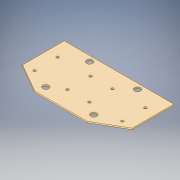
# Autodesk Inventor part: DPLX_P023 Spark Gap Shielding Bottom
Saved by Autodesk Inventor 2018 (Build 220112000, 112)
## iProperties
Created: 2017-11-28
Part Number: DPLX_P023 Spark Gap Shielding Bottom
Material: Polyethylene, High Density
Document SubType Name: Modeling
Designer: Sam
Density: 0.952 g/cm^3
Appearance: Smooth - Off-White
Mass: 11.185 g
Surface Area: 162.174 cm^2
Volume: 11.749 cm^3
Author: Sam
Comments: http://www.eplastics.com/Plastic/G9-G10-FR4-glass-epoxy-sheet/G10NAT-060X12X12
Autodesk Inventor part; units mm, degrees
ref_plane "YZ Plane" through (0, 0, 0) normal (1, 0, 0) x (0, 1, 0)
ref_plane "XZ Plane" through (0, 0, 0) normal (0, 1, 0) x (-1, 0, 0)
ref_plane "XY Plane" through (0, 0, 0) normal (0, 0, 1) x (1, 0, 0)
sketch "Sketch1" plane through (0, 0, 0) normal (0, 1, 0) x (-1, 0, 0)
  line L0 (-63.5, 33.655) -> (63.5, 33.655)
  line L1 (63.5, 33.655) -> (63.5, -33.655)
  line L2 (63.5, -33.655) -> (-63.5, -33.655)
  line L3 (-63.5, -33.655) -> (-63.5, 33.655)
  line L4 (-63.5, 33.655) -> (63.5, -33.655) construction
  line L5 (63.5, 33.655) -> (-63.5, -33.655) construction
  point P0 (0, 0)
  dimension "d0" = 127
  dimension "d1" = 67.31
  constraints: 12 end point, 2 midpoint, 2 parallel, 1 horizontal, 1 perpendicular
  measures "d0" distance of L1.end L2.end
  measures "d1" distance of L0.end L1.end
extrude "Extrusion1" add sketch "Sketch1" along normal mid plane 1.524
sketch "Sketch2" plane through (0, 0.762, 0) normal (0, 1, 0) x (1, 0, 0)
  line L0 (63.5, 33.655) -> (-63.5, 33.655) projected
  line L1 (-63.5, -33.655) -> (63.5, -33.655) projected
  line L2 (-63.5, 33.655) -> (-63.5, -33.655) projected
  line L3 (63.5, -33.655) -> (63.5, 33.655) projected
  point P0 (0, 0)
  point P1 (-50.8, 13.335)
  point P2 (-12.7, 13.335)
  point P3 (12.7, 13.335)
  point P4 (50.8, 13.335)
  point P5 (50.8, -13.335)
  point P6 (12.7, -13.335)
  point P7 (-12.7, -13.335)
  point P8 (-50.8, -13.335)
  point P9 (-50.8, -33.655)
  point P10 (50.8, -33.655)
  point P11 (-63.5, -20.955)
  point P12 (63.5, -20.955)
  dimension "d5" = 20.32
  dimension "d6" = 20.32
  dimension "d7" = 12.7
  dimension "d8" = 50.8
  dimension "d9" = 12.7
  dimension "d10" = 50.8
  constraints: 6 horizontal alignment, 4 vertical alignment
  measures "d5" distance from line of L0 point (-50.8, 13.335)
  measures "d6" distance from line of point (-50.8, -13.335) L1
  measures "d7" distance from line of L2 point (-50.8, 13.335)
  measures "d8" distance from line of point (-12.7, 13.335) L2
  measures "d9" distance from line of point (50.8, 13.335) L3
  measures "d10" distance from line of point (12.7, 13.335) L3
hole "Hole1" at (-50.8, 0.762, -13.335) at (-12.7, 0.762, -13.335) at (12.7, 0.762, -13.335) at (50.8, 0.762, -13.335) at (50.8, 0.762, 13.335) at (12.7, 0.762, 13.335) at (-12.7, 0.762, 13.335) at (-50.8, 0.762, 13.335) direction (0, -1, 0) diameter 3 depth 25.4 tip angle 118
chamfer "Chamfer1" distance 19.05 angle 60 1 edges at (-63.5, 0, 33.655) measured on face at (-63.5, -0.254, 11.2183)
sketch "Sketch4" plane through (0, -0.762, 0) normal (0, -1, 0) x (1, 0, 0)
  circle A0 centre (-27.7751, -27.4042) radius 1.7018
  circle A1 centre (-27.7751, 23.3958) radius 1.7018
  circle A2 centre (27.7749, 23.3958) radius 1.7018
  circle A3 centre (27.7749, -27.4042) radius 1.7018
  point P0 (0, 0)
  constraints: 4 centre point, 8 other
hole "Hole3" at (-27.7751, -0.762, -27.4042) at (-27.7751, -0.762, 23.3958) at (27.7749, -0.762, 23.3958) at (27.7749, -0.762, -27.4042) direction (0, 1, 0) diameter 7 end through all
chamfer "Chamfer2" distance 19.05 angle 60 1 edges at (63.5, 0, 33.655) measured on face at (63.5, 0.254, 11.2183)
equation "\"d6\" = d5"
equation "\"d9\" = d7"
equation "\"d10\" = d8"
body "Solid1"
